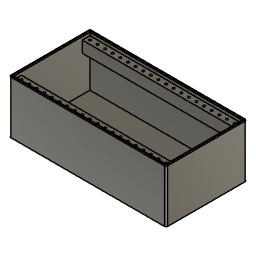
ModularCase v4 (Autodesk Fusion 360 design; units mm, degrees)
Autodesk Fusion 360 part; units mm, degrees
sketch "Sketch1" plane through (0, 0, 0) normal (0, 0, 1) x (1, 0, 0)
  line L0 (0, 0) -> (200, 0)
  line L1 (200, 0) -> (200, 100)
  line L2 (200, 100) -> (0, 100)
  line L3 (0, 100) -> (0, 0)
  line L4 (-3, -3) -> (203, -3)
  line L5 (203, -3) -> (203, 103)
  line L6 (203, 103) -> (-3, 103)
  line L7 (-3, 103) -> (-3, -3)
  line L8 (0, 100) -> (0, 103)
  line L9 (0, 0) -> (0, -3)
  line L10 (200, 0) -> (200, -3)
  line L11 (200, 100) -> (200, 103)
  circle A0 centre (5, 95) radius 1.5
  line L12 (0, 90) -> (200, 90)
  line L13 (0, 10) -> (200, 10)
  circle A1 centre (15, 95) radius 1.5
  circle A2 centre (25, 95) radius 1.5
  circle A3 centre (35, 95) radius 1.5
  circle A4 centre (45, 95) radius 1.5
  circle A5 centre (55, 95) radius 1.5
  circle A6 centre (65, 95) radius 1.5
  circle A7 centre (75, 95) radius 1.5
  circle A8 centre (85, 95) radius 1.5
  circle A9 centre (95, 95) radius 1.5
  circle A10 centre (105, 95) radius 1.5
  circle A11 centre (115, 95) radius 1.5
  circle A12 centre (125, 95) radius 1.5
  circle A13 centre (135, 95) radius 1.5
  circle A14 centre (145, 95) radius 1.5
  circle A15 centre (5, 5) radius 1.5
  circle A16 centre (15, 5) radius 1.5
  circle A17 centre (25, 5) radius 1.5
  circle A18 centre (35, 5) radius 1.5
  circle A19 centre (45, 5) radius 1.5
  circle A20 centre (55, 5) radius 1.5
  circle A21 centre (65, 5) radius 1.5
  circle A22 centre (75, 5) radius 1.5
  circle A23 centre (85, 5) radius 1.5
  circle A24 centre (95, 5) radius 1.5
  circle A25 centre (105, 5) radius 1.5
  circle A26 centre (115, 5) radius 1.5
  circle A27 centre (125, 5) radius 1.5
  circle A28 centre (135, 5) radius 1.5
  circle A29 centre (145, 5) radius 1.5
  circle A30 centre (155, 95) radius 1.5
  circle A31 centre (165, 95) radius 1.5
  circle A32 centre (175, 95) radius 1.5
  circle A33 centre (185, 95) radius 1.5
  circle A34 centre (195, 95) radius 1.5
  circle A35 centre (155, 5) radius 1.5
  circle A36 centre (165, 5) radius 1.5
  circle A37 centre (175, 5) radius 1.5
  circle A38 centre (185, 5) radius 1.5
  circle A39 centre (195, 5) radius 1.5
  dimension "d1" = 3
  dimension "d2" = 3
  dimension "d5" = 190
  dimension "d6" = -90
  dimension "d23" = 200
  dimension "d33" = 100
  constraint horizontal L0
  constraint vertical L1
  constraint horizontal L2
  constraint vertical L3
  constraint coincident L0.start L3.end
  constraint coincident L6 L8.end
  constraint perpendicular L6 L8
  constraint coincident L4 L9.end
  constraint perpendicular L4 L9
  constraint coincident L4 L10.end
  constraint perpendicular L4 L10
  constraint coincident L6 L11.end
  constraint perpendicular L6 L11
  constraint coincident L3 L12.start
  constraint coincident L1 L12.end
  constraint perpendicular L1 L12
  constraint coincident L3 L13.start
  constraint coincident L1 L13.end
  constraint perpendicular L1 L13
  measures "d2" diameter of A0
  measures "d23" distance of L13.start L13.end
  measures "d33" distance of L0 L2
extrude "Extrude1" add sketch "Sketch1" along normal blind 15 from surface at 50 contours L0 L1 L3 L13 | L3 L4 L6 L7 L8 L9 | L0 L4 L9 L10 | L1 L4 L5 L6 L10 L11 | L1 L2 L3 L12 | L2 L6 L8 L11 makes body 1
extrude "Extrude2" add sketch "Sketch1" along normal blind 3 separate body contours L0 L1 L3 L13 | L3 L4 L6 L7 L8 L9 | L0 L4 L9 L10 | L1 L4 L5 L6 L10 L11 | L1 L3 L12 L13 | L1 L2 L3 L12 | L2 L6 L8 L11 | A0 | A1 | A2 | A3 | A4 | A5 | A6 | A7 | A8 | A9 | A10 | A11 | A12 | A13 | A14 | A15 | A16 | A17 | A18 | A19 | A20 | A21 | A22 | A23 | A24 | A25 | A26 | A27 | A28 | A29 | A30 | A31 | A32 | A33 | A34 | A35 | A36 | A37 | A38 | A39 makes body 2
extrude "Extrude3" add sketch "Sketch1" along normal blind 50 contours L3 L4 L6 L7 L8 L9 | L0 L4 L9 L10 | L1 L4 L5 L6 L10 L11 | L2 L6 L8 L11 bodies 1 2
sketch "Sketch2" plane through (0, 0, 0) normal (1, 0, 0) x (0, 1, 0)
  line L0 (90, 50) -> (90, 65)
  line L1 (90, 65) -> (10, 65)
  line L2 (10, 65) -> (10, 50)
  line L3 (10, 50) -> (0, 50)
  line L4 (0, 50) -> (0, 3)
  line L5 (0, 3) -> (100, 3)
  line L6 (100, 3) -> (100, 50)
  line L7 (100, 50) -> (90, 50)
  line L8 (90, 50) -> (100, 40)
  line L9 (10, 50) -> (0, 40)
  line L10 (103, 0) -> (-3, 0)
  dimension "d34" = 40
  constraint coincident L0.start L7.end
  constraint coincident L6 L8.end
  constraint coincident L2.end L3.start
  constraint coincident L4 L9.end
  constraint perpendicular L8 L9
  measures "d34" distance of L9.end L10
extrude "Extrude4" add sketch "Sketch2" along normal up to surface (200 mm away) contours L6 L7 L8 | L3 L4 L9 bodies 1
extrude "Extrude5" add sketch "Sketch1" along normal blind 5 from surface at 65 contours L3 L4 L6 L7 L8 L9 | L0 L4 L9 L10 | L1 L4 L5 L6 L10 L11 | L2 L6 L8 L11 bodies 1
fillet "Fillet1" radius 2 4 edges at (-3, -3, 35) (203, 103, 35) (203, -3, 35) (-3, 103, 35) on bodies 1
fillet "Fillet2" radius 1 12 edges at (-2.4142, 102.4142, 70) (-3, 50, 70) (-2.4142, -2.4142, 70) (100, -3, 70) (202.4142, -2.4142, 70) (203, 50, 70) (202.4142, 102.4142, 70) (100, 103, 70) (100, 100, 70) (0, 50, 70) (100, 0, 70) (200, 50, 70) on bodies 1
equation "d7 = depth - 20 mm"
equation "d12 = depth - 20 mm"
equation "d16 = depth - 5 mm"
equation "d23 = width"
equation "width = ( userWidth * 1 ) * 1 mm"
equation "userWidth = 200" comment "Enter value in mm"
equation "holeAmount = userWidth / 10"
equation "userDepth = 70"
equation "userHeight = 100"
equation "depth = ( userDepth * 1 ) * 1 mm"
equation "height = ( userHeight * 1 ) * 1 mm"
equation "d34 = depth - 30 mm"
